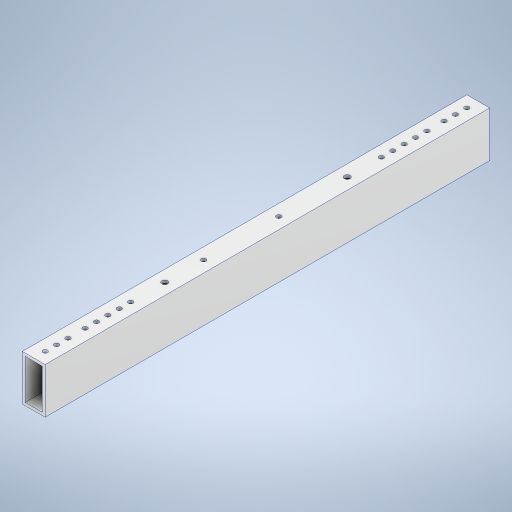
# Autodesk Inventor part: (1)alum_swerve_bar
Saved by Autodesk Inventor 2024 (Build 280153000, 153)
## iProperties
Created: 2023-10-09
Part Number: (1)alum_swerve_bar
Material: Aluminum 6061
Document SubType Name: Modeling
Designer: s137416
Density: 2.7 g/cm^3
Appearance: Aluminum - Flat
Author: s137416
Autodesk Inventor part; units mm, degrees
ref_plane "YZ Plane" through (0, 0, 0) normal (1, 0, 0) x (0, 1, 0)
ref_plane "XZ Plane" through (0, 0, 0) normal (0, 1, 0) x (-1, 0, 0)
ref_plane "XY Plane" through (0, 0, 0) normal (0, 0, 1) x (1, 0, 0)
sketch "Sketch1" plane through (0, 0, 0) normal (0, 1, 0) x (-1, 0, 0)
  line L0 (6.9765, 470.5322) -> (-18.4235, 470.5322)
  line L1 (-18.4235, 470.5322) -> (-18.4235, -24.7678)
  line L2 (-18.4235, -24.7678) -> (6.9765, -24.7678)
  line L3 (6.9765, -24.7678) -> (6.9765, 470.5322)
  circle A0 centre (-5.7235, 457.8322) radius 2.5019
  circle A1 centre (-5.7235, 445.1322) radius 2.5019
  circle A2 centre (-5.7235, 432.4322) radius 2.5019
  circle A3 centre (-5.7235, 413.3822) radius 2.5019
  circle A4 centre (-5.7235, 400.6822) radius 2.5019
  circle A5 centre (-5.7235, 387.9822) radius 2.5019
  circle A6 centre (-5.7235, 400.6822) radius 2.5019
  circle A7 centre (-5.7235, 375.2822) radius 2.5019
  circle A8 centre (-5.7235, 362.5822) radius 2.5019
  circle A9 centre (-5.7235, -12.0678) radius 2.5019
  circle A10 centre (-5.7235, 0.6322) radius 2.5019
  circle A11 centre (-5.7235, 13.3322) radius 2.5019
  circle A12 centre (-5.7235, 32.3822) radius 2.5019
  circle A13 centre (-5.7235, 45.0822) radius 2.5019
  circle A14 centre (-5.7235, 57.7822) radius 2.5019
  circle A15 centre (-5.7235, 70.4822) radius 2.5019
  circle A16 centre (-5.7235, 83.1822) radius 2.5019
  circle A17 centre (-5.7235, 164.4368) radius 2.5527
  circle A18 centre (-5.7235, 281.3276) radius 2.5527
  point P0 (0, 0)
  dimension "d0" = 25.4
  dimension "d1" = 495.3
  dimension "d2" = 5.0038
  dimension "d3" = 5.0038
  dimension "d4" = 5.0038
  dimension "d5" = 5.0038
  dimension "d6" = 5.0038
  dimension "d7" = 5.0038
  dimension "d8" = 5.0038
  dimension "d9" = 5.0038
  dimension "d10" = 12.7
  dimension "d11" = 12.7
  dimension "d12" = 12.7
  dimension "d13" = 57.15
  dimension "d14" = 12.7
  dimension "d15" = 12.7
  dimension "d16" = 12.7
  dimension "d17" = 12.7
  dimension "d18" = 5.0038
  dimension "d19" = 12.7
  dimension "d20" = 5.0038
  dimension "d21" = 5.0038
  dimension "d22" = 5.0038
  dimension "d23" = 12.7
  dimension "d24" = 12.7
  dimension "d25" = 12.7
  dimension "d26" = 5.0038
  dimension "d27" = 5.0038
  dimension "d28" = 5.0038
  dimension "d29" = 5.0038
  dimension "d30" = 5.0038
  dimension "d31" = 57.15
  dimension "d32" = 12.7
  dimension "d33" = 12.7
  dimension "d34" = 12.7
  dimension "d35" = 12.7
  dimension "d52" = 5.1054
  dimension "d53" = 5.1054
  dimension "d54" = 76.2
  dimension "d55" = 76.2
  constraints: 19 centre point, 8 end point, 2 parallel, 1 horizontal, 1 perpendicular
  measures "d0" distance of L2.end L1.end
  measures "d1" distance of L2.end L0.start
  measures "d2" diameter of A0
  measures "d3" diameter of A1
  measures "d4" diameter of A2
  measures "d5" diameter of A3
  measures "d6" diameter of A4
  measures "d7" diameter of A5
  measures "d8" diameter of A6
  measures "d9" diameter of A7
  measures "d10" distance from line of L0 A0.centre
  measures "d11" distance of A0.centre A1.centre
  measures "d12" distance of A1.centre A2.centre
  measures "d13" distance from line of L0 A3.centre
  measures "d14" distance of A3.centre A4.centre
  measures "d15" distance of A4.centre A5.centre
  measures "d16" distance of A6.centre A5.centre
  measures "d17" distance of A5.centre A7.centre
  measures "d18" diameter of A8
  measures "d19" distance of A7.centre A8.centre
  measures "d20" diameter of A9
  measures "d21" diameter of A10
  measures "d22" diameter of A11
  measures "d23" distance from line of L2 A9.centre
  measures "d24" distance of A10.centre A9.centre
  measures "d25" distance of A11.centre A10.centre
  measures "d26" diameter of A12
  measures "d27" diameter of A13
  measures "d28" diameter of A14
  measures "d29" diameter of A15
  measures "d30" diameter of A16
  measures "d31" distance from line of L2 A12.centre
  measures "d32" distance of A12.centre A13.centre
  measures "d33" distance of A13.centre A14.centre
  measures "d34" distance of A14.centre A15.centre
  measures "d35" distance of A15.centre A16.centre
  measures "d52" diameter of A17
  measures "d53" diameter of A18
extrude "Extrusion1" add sketch "Sketch1" along normal blind 50.8 contours L3 L2 L1 L0 | A17 | A18
shell "Shell2" thickness 3.175 removed faces 17 at (1.4901, 33.8667, 470.5322) at (4.6509, 33.8667, 460.0925) at (6.796, 33.8667, 377.5425) at (8.0251, 16.9333, 84.1628) at (3.2297, 33.8667, -12.2692) at (8.0251, 16.9333, 71.4628) at (4.6509, 33.8667, 447.3925) at (3.9903, 33.8667, 430.6278) at (3.9903, 33.8667, 411.5778) at (4.6509, 33.8667, 402.9425) at (3.4218, 33.8667, 387.0015) at (3.2297, 33.8667, 362.3808) at (3.2297, 33.8667, 57.5808) at (3.2297, 33.8667, 44.8808) at (3.2297, 33.8667, 32.1808) at (3.2297, 33.8667, 13.1308) at (3.2297, 33.8667, 0.4308)
shell "Shell3" thickness 3.175 removed faces 2 at (9.9568, 33.8667, -24.7678) at (8.8985, 17.9917, -21.5928)
sketch "Sketch2" plane through (0, 50.8, 0) normal (0, 1, 0) x (1, 0, 0)
  circle A0 centre (5.7235, -324.4822) radius 3.175
  line L0 (-6.9765, -470.5322) -> (18.4235, -470.5322) projected
  circle A1 centre (5.7235, -121.2822) radius 3.175
  line L1 (18.4235, 24.7678) -> (-6.9765, 24.7678) projected
  point P0 (0, 0)
  dimension "d41" = 6.35
  dimension "d42" = 146.05
  dimension "d43" = 6.35
  dimension "d44" = 146.05
  constraints: 2 centre point
  measures "d41" diameter of A0
  measures "d42" distance from line of L0 A0.centre
  measures "d43" diameter of A1
  measures "d44" distance from line of L1 A1.centre
hole "Hole1" at (5.7235, 50.8, 324.4822) at (5.7235, 50.8, 121.2822) direction (0, -1, 0) diameter 6.35 end through all
sketch "Sketch3" plane through (0, 50.8, 0) normal (0, 1, 0) x (1, 0, 0)
  circle A0 centre (5.7235, -281.3276) radius 2.5527
  circle A1 centre (5.7235, -362.5822) radius 2.5019 projected
  circle A2 centre (5.7235, -197.4822) radius 2.5527
  circle A3 centre (5.7235, -121.2822) radius 3.175 projected
  point P0 (0, 0)
  dimension "d56" = 5.1054
  dimension "d57" = 76.2
  dimension "d58" = 5.1054
  dimension "d59" = 76.2
  constraints: 2 centre point
  measures "d56" diameter of A0
  measures "d58" diameter of A2
  measures "d59" distance of A3.centre A2.centre
hole "Hole2" at (5.7235, 50.8, 281.3276) at (5.7235, 50.8, 197.4822) direction (0, -1, 0) diameter 5.1054 end through all
body "Solid1"
